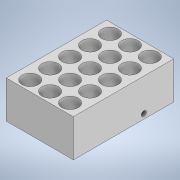
# Autodesk Inventor part: Thermal_topplate_5mL
Saved by Autodesk Inventor 2020 (Build 240168000, 168)
## iProperties
Created: 2021-08-09
Part Number: Thermal_topplate_5mL
Material: Generic
Document SubType Name: Modeling
Designer: pab2
Density: 1 g/cm^3
Appearance: Default
Author: pab2
Autodesk Inventor part; units mm, degrees
ref_plane "YZ Plane" through (0, 0, 0) normal (1, 0, 0) x (0, 1, 0)
ref_plane "XZ Plane" through (0, 0, 0) normal (0, 1, 0) x (-1, 0, 0)
ref_plane "XY Plane" through (0, 0, 0) normal (0, 0, 1) x (1, 0, 0)
sketch "Sketch1" plane through (0, 0, 0) normal (0, 1, 0) x (-1, 0, 0)
  line L0 (0, 0) -> (85.48, 0)
  line L1 (85.48, 0) -> (85.48, -127.76)
  line L2 (85.48, -127.76) -> (0, -127.76)
  line L3 (0, -127.76) -> (0, 0)
  line L4 (85.48, 0) -> (67.5195, -17.9605)
  line L5 (85.48, 0) -> (110.88, 0) construction
  line L6 (0, 0) -> (17.9605, -17.9605)
  line L7 (85.48, -127.76) -> (67.5195, -109.7995)
  line L8 (85.48, -127.76) -> (110.88, -127.76) construction
  line L9 (0, -127.76) -> (17.9605, -109.7995)
  line L10 (0, -127.76) -> (25.4, -127.76) construction
  dimension "d0" = 85.48
  dimension "d1" = 127.76
  dimension "d2" = 25.4
  dimension "d3" = 135
  dimension "d4" = 25.4
  dimension "d5" = 25.4
  dimension "d6" = 135
  dimension "d7" = 25.4
  dimension "d8" = 45
  constraints: 22 end point, 4 horizontal, 3 equal length, 2 parallel, 1 perpendicular
  measures "d0" distance of L1.end L2.end
  measures "d1" distance of L0.end L1.end
  measures "d2" distance of L0.end L4.end
  measures "d3" angle of L4 L5
  measures "d4" distance of L0.start L6.end
  measures "d5" distance of L1.end L7.end
  measures "d6" angle of L8 L7
  measures "d7" distance of L2.end L9.end
  measures "d8" angle of L10 L9
extrude "Extrusion1" add sketch "Sketch1" along normal blind 47.7
sketch "Sketch2" plane through (0, 0, 0) normal (0, -1, 0) x (1, 0, 0)
  line L0 (-85.48, 0) -> (0, 0) projected
  line L1 (0, 0) -> (-17.9605, -17.9605)
  line L2 (0, 0) -> (25.4, 0) construction
  line L3 (0, 0) -> (0, -127.76) projected
  line L4 (0, -127.76) -> (-17.9605, -109.7995)
  line L5 (0, -127.76) -> (25.4, -127.76) construction
  line L6 (-85.48, -127.76) -> (-85.48, 0) projected
  line L7 (-85.48, 0) -> (-67.5195, -17.9605)
  line L8 (-85.48, 0) -> (-60.08, 0) construction
  line L9 (0, -127.76) -> (-85.48, -127.76) projected
  line L10 (-85.48, -127.76) -> (-67.5195, -109.7995)
  line L11 (-85.48, -127.76) -> (-60.08, -127.76) construction
  dimension "d11" = 25.4
  dimension "d12" = 135
  dimension "d13" = 25.4
  dimension "d14" = 135
  dimension "d15" = 25.4
  dimension "d16" = 45
  dimension "d17" = 25.4
  dimension "d18" = 45
  constraints: 16 end point, 4 equal length, 4 horizontal
  measures "d11" distance of L0.end L1.end
  measures "d12" angle of L1 L2
  measures "d13" distance of L3.end L4.end
  measures "d14" angle of L5 L4
  measures "d15" distance of L0.start L7.end
  measures "d16" angle of L7 L8
  measures "d17" distance of L6.start L10.end
  measures "d18" angle of L11 L10
hole "Hole1" at (-17.9605, 0, -17.9605) at (-67.5195, 0, -17.9605) at (-67.5195, 0, -109.7995) at (-17.9605, 0, -109.7995) direction (0, 1, 0) diameter 3.683 depth 9.525 tip angle 118 thread size "10-24 UNC" class "2B" standard "ANSI Unified Screw Threads"
sketch "Sketch4" plane through (0, 47.7, 0) normal (0, 1, 0) x (1, 0, 0)
  line L0 (0, -1.0521) -> (19.05, -1.0521) construction
  line L1 (0, 0) -> (0, 127.76) projected
  line L2 (0, 18.3507) -> (0, 0)
  line L3 (0, 0) -> (-18.7946, 0)
  line L4 (0, 0) -> (-17.3355, 0)
  line L5 (-17.3355, 0) -> (-17.3355, 13.1191)
  line L6 (-17.3355, 13.1191) -> (0, 13.1191)
  line L7 (0, 13.1191) -> (0, 0)
  dimension "d41" = 17.3355
  dimension "d42" = 13.1191
  constraints: 14 end point, 2 horizontal, 2 parallel, 1 perpendicular
  measures "d41" distance of L5.end L6.end
  measures "d42" distance of L4.end L5.end
hole "Hole2" at (-17.3355, 47.7, -13.1191) direction (0, -1, 0) diameter 21 depth 35
pattern_linear "Rectangular Pattern1" count 3 spacing 25.4 along (-1, 0, 0) count 5 spacing 25.4 along (0, 0, -1) of "Hole2"
sketch "Sketch5" plane through (-85.48, 0, -127.76) normal (-1, 0, 0) x (0, 0, 1)
  line L0 (127.76, 0) -> (127.76, 47.7) projected
  line L1 (127.76, 0) -> (89.66, 0)
  line L2 (89.66, 0) -> (89.66, 6.35)
  line L3 (89.66, 6.35) -> (127.76, 6.35)
  line L4 (127.76, 6.35) -> (127.76, 0)
  line L5 (62.646, 6.35) -> (127.76, 6.35)
  line L6 (127.76, 6.35) -> (127.76, 0)
  line L7 (127.76, 0) -> (62.646, 0)
  line L8 (62.646, 0) -> (62.646, 6.35)
  dimension "d43" = 38.1
  dimension "d44" = 6.35
  constraints: 16 end point, 4 parallel, 2 horizontal, 2 perpendicular, 1 point on line
  measures "d43" distance of L2.end L3.end
  measures "d44" distance of L1.end L2.end
hole "Hole3" at (-85.48, 6.35, -38.1) direction (1, 0, 0) diameter 6.35 depth 31.75 tip angle 118
sketch "Sketch6" plane through (-85.48, 0, -127.76) normal (-1, 0, 0) x (0, 0, 1)
  line L0 (61.854, 6.5465) -> (127.76, 6.5465)
  line L1 (127.76, 6.5465) -> (127.76, 0.1965)
  line L2 (127.76, 0.1965) -> (61.854, 0.1965)
  line L3 (61.854, 0.1965) -> (61.854, 6.5465)
  point P0 (127.76, 0)
  dimension "d52" = 6.35
  constraints: 8 end point, 2 parallel, 1 horizontal, 1 perpendicular
  measures "d52" distance of L0.end L1.end
hole "Hole4" at (-85.48, 6.5465, -65.906) direction (1, 0, 0) diameter 3.175 depth 50.8 tip angle 118
sketch "Sketch7" plane through (0, 0, 0) normal (1, 0, 0) x (0, 0, -1)
  line L0 (127.76, 0) -> (0, 0) projected
  line L1 (127.76, 0) -> (89.66, 0)
  line L2 (89.66, 0) -> (89.66, 6.35)
  line L3 (89.66, 6.35) -> (127.76, 6.35)
  line L4 (127.76, 6.35) -> (127.76, 0)
  dimension "d60" = 38.1
  dimension "d61" = 6.35
  constraints: 8 end point, 2 parallel, 1 horizontal, 1 perpendicular
  measures "d60" distance of L2.end L3.end
  measures "d61" distance of L1.end L2.end
hole "Hole5" at (0, 6.35, -89.66) direction (-1, 0, 0) diameter 6.35 depth 31.75 tip angle 118
body "Solid1"
